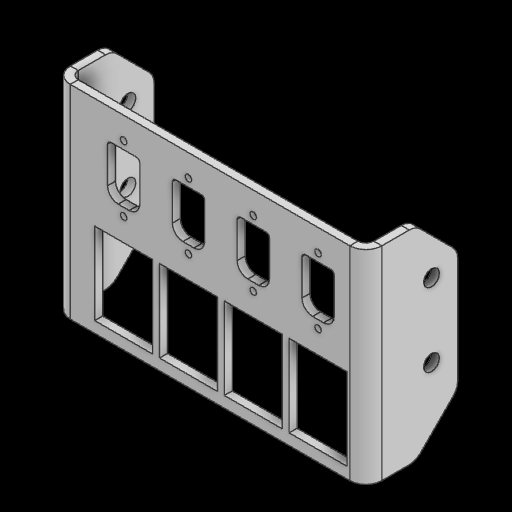
# Autodesk Inventor part: PowerHubFrontPanel
Saved by Autodesk Inventor 2025.2 (Build 292293000, 293)
## iProperties
Created: 2026-06-06
Part Number: PowerHubFrontPanel
Material: Generic
Document SubType Name: Sheet Metal
Designer: valer
Density: 1 g/cm^3
Appearance: Default
Sheet Metal Rule: Default
Author: valer
Autodesk Inventor part; units mm, degrees
ref_plane "YZ Plane" through (0, 0, 0) normal (1, 0, 0) x (0, 1, 0)
ref_plane "XZ Plane" through (0, 0, 0) normal (0, 1, 0) x (-1, 0, 0)
ref_plane "XY Plane" through (0, 0, 0) normal (0, 0, 1) x (1, 0, 0)
sketch "Base" plane through (0, 0, 0) normal (0, 0, 1) x (1, 0, 0)
  line L0 (-44.957, 34.75) -> (-28.957, 34.75) construction
  line L1 (-28.957, 34.75) -> (-28.957, 0.75) construction
  line L2 (-28.957, 0.75) -> (-44.957, 0.75) construction
  line L3 (-44.957, 0.75) -> (-44.957, 34.75) construction
  line L4 (-49.276, -3.25) -> (-24.638, -3.25) construction
  line L5 (-24.638, -3.25) -> (-24.638, -34.75) construction
  line L6 (-24.638, -34.75) -> (-49.276, -34.75) construction
  line L7 (-49.276, -34.75) -> (-49.276, -3.25) construction
  line L8 (-36.957, 0.75) -> (-36.957, -3.25) construction
  line L9 (-20.319, 0.75) -> (-20.319, 34.75) construction
  line L10 (-20.319, 34.75) -> (-4.319, 34.75) construction
  line L11 (-4.319, 34.75) -> (-4.319, 0.75) construction
  line L12 (-4.319, 0.75) -> (-20.319, 0.75) construction
  line L13 (-24.638, -3.25) -> (0, -3.25) construction
  line L14 (-24.638, -34.75) -> (-24.638, -3.25) construction
  line L15 (0, -3.25) -> (0, -34.75) construction
  line L16 (0, -34.75) -> (-24.638, -34.75) construction
  line L17 (4.319, 0.75) -> (4.319, 34.75) construction
  line L18 (4.319, 34.75) -> (20.319, 34.75) construction
  line L19 (20.319, 34.75) -> (20.319, 0.75) construction
  line L20 (20.319, 0.75) -> (4.319, 0.75) construction
  line L21 (0, -3.25) -> (24.638, -3.25) construction
  line L22 (0, -34.75) -> (0, -3.25) construction
  line L23 (24.638, -3.25) -> (24.638, -34.75) construction
  line L24 (24.638, -34.75) -> (0, -34.75) construction
  line L25 (28.957, 0.75) -> (28.957, 34.75) construction
  line L26 (28.957, 34.75) -> (44.957, 34.75) construction
  line L27 (44.957, 34.75) -> (44.957, 0.75) construction
  line L28 (44.957, 0.75) -> (28.957, 0.75) construction
  line L29 (24.638, -3.25) -> (49.276, -3.25) construction
  line L30 (24.638, -34.75) -> (24.638, -3.25) construction
  line L31 (49.276, -3.25) -> (49.276, -34.75) construction
  line L32 (49.276, -34.75) -> (24.638, -34.75) construction
  line L33 (-53.276, 38.75) -> (53.276, 38.75)
  line L34 (53.276, 38.75) -> (53.276, -38.75)
  line L35 (53.276, -38.75) -> (-53.276, -38.75)
  line L36 (-53.276, -38.75) -> (-53.276, 38.75)
  line L37 (0, -54.25) -> (0, 54.25)
  line L38 (-53.276, 38.75) -> (53.276, -38.75) construction
  point P0 (-12.319, 0.75)
  point P1 (-12.319, -3.25)
  point P2 (12.319, 0.75)
  point P3 (12.319, -3.25)
  point P4 (36.957, 0.75)
  point P5 (36.957, -3.25)
  point P6 (0, 0)
  point P7 (0, 0)
  dimension "d103" = 16
  dimension "d104" = 34
  dimension "d105" = 24.638
  dimension "d106" = 31.5
  dimension "d107" = 4
  dimension "d110" = 24.638
  dimension "d125" = 4
  dimension "d126" = 4
  dimension "d131" = 4
  dimension "d132" = 4
  measures "d103" distance of L0.start L0.end
  measures "d104" distance of L0.end L1.end
  measures "d105" distance of L5.end L6.end
  measures "d106" distance of L4.end L5.end
  measures "d107" distance between parallel lines of L4 L2
  measures "d110" distance of L2.end L9.start
  measures "d125" distance between parallel lines of L36 L7
  measures "d126" distance between parallel lines of L34 L31
  measures "d131" distance between parallel lines of L33 L26
  measures "d132" distance between parallel lines of L35 L32
extrude "Plate1" add sketch "Base" along normal blind 3.048
sketch "Instruments" plane through (0, 0, 0) normal (0, 0, -1) x (-1, 0, 0)
  circle A0 centre (-41.1741, 14.35) radius 2.5 construction
  circle A1 centre (-41.1741, 21.35) radius 2.5 construction
  arc A2 (-47.0741, 12.4) -> (-43.2741, 8.6) centre (-43.2741, 12.4) ccw construction
  line L0 (-43.2741, 8.6) -> (-39.0741, 8.6) construction
  arc A3 (-39.0741, 8.6) -> (-35.2741, 12.4) centre (-39.0741, 12.4) ccw construction
  line L1 (-35.2741, 12.4) -> (-35.2741, 26.1) construction
  arc A4 (-35.2741, 26.1) -> (-36.2741, 27.1) centre (-36.2741, 26.1) ccw construction
  line L2 (-36.2741, 27.1) -> (-46.0741, 27.1) construction
  arc A5 (-46.0741, 27.1) -> (-47.0741, 26.1) centre (-46.0741, 26.1) ccw construction
  line L3 (-47.0741, 26.1) -> (-47.0741, 12.4) construction
  circle A6 centre (-16.4741, 14.35) radius 2.5 construction
  circle A7 centre (-16.4741, 21.35) radius 2.5 construction
  arc A8 (-22.3741, 12.4) -> (-18.5741, 8.6) centre (-18.5741, 12.4) ccw construction
  line L4 (-18.5741, 8.6) -> (-14.3741, 8.6) construction
  arc A9 (-14.3741, 8.6) -> (-10.5741, 12.4) centre (-14.3741, 12.4) ccw construction
  line L5 (-10.5741, 12.4) -> (-10.5741, 26.1) construction
  arc A10 (-10.5741, 26.1) -> (-11.5741, 27.1) centre (-11.5741, 26.1) ccw construction
  line L6 (-11.5741, 27.1) -> (-21.3741, 27.1) construction
  arc A11 (-21.3741, 27.1) -> (-22.3741, 26.1) centre (-21.3741, 26.1) ccw construction
  line L7 (-22.3741, 26.1) -> (-22.3741, 12.4) construction
  circle A12 centre (8.2259, 14.35) radius 2.5 construction
  circle A13 centre (8.2259, 21.35) radius 2.5 construction
  arc A14 (2.3259, 12.4) -> (6.1259, 8.6) centre (6.1259, 12.4) ccw construction
  line L8 (6.1259, 8.6) -> (10.3259, 8.6) construction
  arc A15 (10.3259, 8.6) -> (14.1259, 12.4) centre (10.3259, 12.4) ccw construction
  line L9 (14.1259, 12.4) -> (14.1259, 26.1) construction
  arc A16 (14.1259, 26.1) -> (13.1259, 27.1) centre (13.1259, 26.1) ccw construction
  line L10 (13.1259, 27.1) -> (3.3259, 27.1) construction
  arc A17 (3.3259, 27.1) -> (2.3259, 26.1) centre (3.3259, 26.1) ccw construction
  line L11 (2.3259, 26.1) -> (2.3259, 12.4) construction
  circle A18 centre (32.9259, 14.35) radius 2.5 construction
  circle A19 centre (32.9259, 21.35) radius 2.5 construction
  arc A20 (27.0259, 12.4) -> (30.8259, 8.6) centre (30.8259, 12.4) ccw construction
  line L12 (30.8259, 8.6) -> (35.0259, 8.6) construction
  arc A21 (35.0259, 8.6) -> (38.8259, 12.4) centre (35.0259, 12.4) ccw construction
  line L13 (38.8259, 12.4) -> (38.8259, 26.1) construction
  arc A22 (38.8259, 26.1) -> (37.8259, 27.1) centre (37.8259, 26.1) ccw construction
  line L14 (37.8259, 27.1) -> (28.0259, 27.1) construction
  arc A23 (28.0259, 27.1) -> (27.0259, 26.1) centre (28.0259, 26.1) ccw construction
  line L15 (27.0259, 26.1) -> (27.0259, 12.4) construction
  line L16 (-47.8197, -7.45) -> (-34.5285, -7.45) construction
  line L17 (-34.5285, -7.45) -> (-34.5285, -30.45) construction
  line L18 (-34.5285, -30.45) -> (-47.8197, -30.45) construction
  line L19 (-47.8197, -30.45) -> (-47.8197, -7.45) construction
  line L20 (-30.3791, -3.6) -> (-51.9691, -3.6) construction
  line L21 (-51.9691, -3.6) -> (-51.9691, -34.3) construction
  line L22 (-51.9691, -34.3) -> (-30.3791, -34.3) construction
  line L23 (-30.3791, -34.3) -> (-30.3791, -3.6) construction
  line L24 (-23.1197, -7.45) -> (-9.8285, -7.45) construction
  line L25 (-9.8285, -7.45) -> (-9.8285, -30.45) construction
  line L26 (-9.8285, -30.45) -> (-23.1197, -30.45) construction
  line L27 (-23.1197, -30.45) -> (-23.1197, -7.45) construction
  line L28 (-5.6791, -3.6) -> (-27.2691, -3.6) construction
  line L29 (-27.2691, -3.6) -> (-27.2691, -34.3) construction
  line L30 (-27.2691, -34.3) -> (-5.6791, -34.3) construction
  line L31 (-5.6791, -34.3) -> (-5.6791, -3.6) construction
  line L32 (1.5803, -7.45) -> (14.8715, -7.45) construction
  line L33 (14.8715, -7.45) -> (14.8715, -30.45) construction
  line L34 (14.8715, -30.45) -> (1.5803, -30.45) construction
  line L35 (1.5803, -30.45) -> (1.5803, -7.45) construction
  line L36 (19.0209, -3.6) -> (-2.5691, -3.6) construction
  line L37 (-2.5691, -3.6) -> (-2.5691, -34.3) construction
  line L38 (-2.5691, -34.3) -> (19.0209, -34.3) construction
  line L39 (19.0209, -34.3) -> (19.0209, -3.6) construction
  line L40 (26.2803, -7.45) -> (39.5715, -7.45) construction
  line L41 (39.5715, -7.45) -> (39.5715, -30.45) construction
  line L42 (39.5715, -30.45) -> (26.2803, -30.45) construction
  line L43 (26.2803, -30.45) -> (26.2803, -7.45) construction
  line L44 (43.7209, -3.6) -> (22.1309, -3.6) construction
  line L45 (22.1309, -3.6) -> (22.1309, -34.3) construction
  line L46 (22.1309, -34.3) -> (43.7209, -34.3) construction
  line L47 (43.7209, -34.3) -> (43.7209, -3.6) construction
  line L48 (-46.0741, 27.35) -> (-36.2741, 27.35)
  arc A24 (-35.0241, 26.1) -> (-36.2741, 27.35) centre (-36.2741, 26.1) ccw
  line L49 (-35.0241, 26.1) -> (-35.0241, 12.4)
  arc A25 (-39.0741, 8.35) -> (-35.0241, 12.4) centre (-39.0741, 12.4) ccw
  line L50 (-39.0741, 8.35) -> (-43.2741, 8.35)
  arc A26 (-47.3241, 12.4) -> (-43.2741, 8.35) centre (-43.2741, 12.4) ccw
  line L51 (-47.3241, 12.4) -> (-47.3241, 26.1)
  arc A27 (-46.0741, 27.35) -> (-47.3241, 26.1) centre (-46.0741, 26.1) ccw
  line L52 (-21.3741, 27.35) -> (-11.5741, 27.35)
  arc A28 (-10.3241, 26.1) -> (-11.5741, 27.35) centre (-11.5741, 26.1) ccw
  line L53 (-10.3241, 26.1) -> (-10.3241, 12.4)
  arc A29 (-14.3741, 8.35) -> (-10.3241, 12.4) centre (-14.3741, 12.4) ccw
  line L54 (-14.3741, 8.35) -> (-18.5741, 8.35)
  arc A30 (-22.6241, 12.4) -> (-18.5741, 8.35) centre (-18.5741, 12.4) ccw
  line L55 (-22.6241, 12.4) -> (-22.6241, 26.1)
  arc A31 (-21.3741, 27.35) -> (-22.6241, 26.1) centre (-21.3741, 26.1) ccw
  line L56 (3.3259, 27.35) -> (13.1259, 27.35)
  arc A32 (14.3759, 26.1) -> (13.1259, 27.35) centre (13.1259, 26.1) ccw
  line L57 (14.3759, 26.1) -> (14.3759, 12.4)
  arc A33 (10.3259, 8.35) -> (14.3759, 12.4) centre (10.3259, 12.4) ccw
  line L58 (10.3259, 8.35) -> (6.1259, 8.35)
  arc A34 (2.0759, 12.4) -> (6.1259, 8.35) centre (6.1259, 12.4) ccw
  line L59 (2.0759, 12.4) -> (2.0759, 26.1)
  arc A35 (3.3259, 27.35) -> (2.0759, 26.1) centre (3.3259, 26.1) ccw
  line L60 (28.0259, 27.35) -> (37.8259, 27.35)
  arc A36 (39.0759, 26.1) -> (37.8259, 27.35) centre (37.8259, 26.1) ccw
  line L61 (39.0759, 26.1) -> (39.0759, 12.4)
  arc A37 (35.0259, 8.35) -> (39.0759, 12.4) centre (35.0259, 12.4) ccw
  line L62 (35.0259, 8.35) -> (30.8259, 8.35)
  arc A38 (26.7759, 12.4) -> (30.8259, 8.35) centre (30.8259, 12.4) ccw
  line L63 (26.7759, 12.4) -> (26.7759, 26.1)
  arc A39 (28.0259, 27.35) -> (26.7759, 26.1) centre (28.0259, 26.1) ccw
  line L64 (43.9709, -3.35) -> (21.8809, -3.35)
  line L65 (21.8809, -3.35) -> (21.8809, -34.55)
  line L66 (21.8809, -34.55) -> (43.9709, -34.55)
  line L67 (43.9709, -34.55) -> (43.9709, -3.35)
  line L68 (-2.8191, -3.35) -> (19.2709, -3.35)
  line L69 (19.2709, -3.35) -> (19.2709, -34.55)
  line L70 (19.2709, -34.55) -> (-2.8191, -34.55)
  line L71 (-2.8191, -34.55) -> (-2.8191, -3.35)
  line L72 (-27.5191, -3.35) -> (-5.4291, -3.35)
  line L73 (-5.4291, -3.35) -> (-5.4291, -34.55)
  line L74 (-5.4291, -34.55) -> (-27.5191, -34.55)
  line L75 (-27.5191, -34.55) -> (-27.5191, -3.35)
  line L76 (-52.2191, -3.35) -> (-30.1291, -3.35)
  line L77 (-30.1291, -3.35) -> (-30.1291, -34.55)
  line L78 (-30.1291, -34.55) -> (-52.2191, -34.55)
  line L79 (-52.2191, -34.55) -> (-52.2191, -3.35)
  circle A40 centre (32.9259, 30.35) radius 1.55 construction
  circle A41 centre (32.9259, 5.35) radius 1.55 construction
  circle A42 centre (8.2259, 5.35) radius 1.55 construction
  circle A43 centre (8.2259, 30.35) radius 1.55 construction
  circle A44 centre (-16.4741, 30.35) radius 1.55 construction
  circle A45 centre (-16.4741, 5.35) radius 1.55 construction
  circle A46 centre (-41.1741, 30.35) radius 1.55 construction
  circle A47 centre (-41.1741, 5.35) radius 1.55 construction
  circle A48 centre (-41.1741, 30.35) radius 1.25
  circle A49 centre (-16.4741, 30.35) radius 1.25
  circle A50 centre (8.2259, 30.35) radius 1.25
  circle A51 centre (32.9259, 30.35) radius 1.25
  circle A52 centre (-41.1741, 5.35) radius 1.25
  circle A53 centre (-16.4741, 5.35) radius 1.25
  circle A54 centre (8.2259, 5.35) radius 1.25
  circle A55 centre (32.9259, 5.35) radius 1.25
  point P0 (0, 0)
  dimension "d134" = 0.25
  dimension "d135" = 0.25
  dimension "d136" = 0.25
  dimension "d137" = 0.25
  dimension "d138" = 0.25
  dimension "d139" = 0.25
  dimension "d140" = 0.25
  dimension "d141" = 0.25
  dimension "d144" = 2.5
  constraints: 64 end point, 32 point on circle, 24 centre point, 8 coincident, 7 equal radius, 40 other
  measures "d134" distance between parallel lines of L2 L48
  measures "d135" distance between parallel lines of L6 L52
  measures "d136" distance between parallel lines of L10 L56
  measures "d137" distance between parallel lines of L14 L60
  measures "d138" distance between parallel lines of L47 L67
  measures "d139" distance between parallel lines of L36 L68
  measures "d140" distance between parallel lines of L28 L72
  measures "d141" distance between parallel lines of L20 L76
  measures "d144" diameter of A48
extrude "InstrumentsFeature" cut sketch "Instruments" against normal blind 3.048
sketch "Sketch10" plane through (-56.324, 38.75, -3.048) normal (-1, 0, 0) x (0, -1, 0)
  line L0 (77.5, 0) -> (0, 0)
  line L1 (0, 0) -> (0, -28.904)
  line L2 (0, -28.904) -> (77.5, -28.904)
  line L3 (77.5, -28.904) -> (77.5, 0)
  constraints: 6 end point, 1 horizontal, 1 perpendicular, 1 vertical
edge flange "MountFeature" height 35 angle 90 thickness 3.048 bend radius 3.048 thickness toward (-1, 0, 0) relief straight relief width 3.048 relief depth 1.524 corner gap 3.048 corner form 0 edges at (-53.276, 0, 0) (53.276, 0, 0) wall of the first edge with corners at (-56.324, -38.75, -3.048) (-56.324, 38.75, -3.048) (-56.324, 38.75, -31.952) (-56.324, -38.75, -31.952)
bend "Bend1"
corner "Corner1"
chamfer "MountChamfersFeature" distance 16 angle 45 4 edges at (57.848, -38.75, -31.952) (-57.848, -38.75, -31.952) (57.848, 38.75, -31.952) (-57.848, 38.75, -31.952)
fillet "MountFilletsFeature" radius 6 8 edges at (57.848, -38.75, -15.952) (57.848, -22.75, -31.952) (-57.848, -38.75, -15.952) (-57.848, -22.75, -31.952) (57.848, 22.75, -31.952) (57.848, 38.75, -15.952) (-57.848, 22.75, -31.952) (-57.848, 38.75, -15.952)
sketch "Sketch11" plane through (-59.372, -38.75, -3.048) normal (-1, 0, 0) x (0, 0, 1)
  circle A0 centre (-18.904, 29.5122) radius 3
  circle A1 centre (-18.904, 57.5122) radius 3
  arc A2 (-16.7827, 31.6335) -> (-21.0253, 27.3909) centre (-18.904, 29.5122) ccw projected
  arc A3 (-16.7827, 59.6335) -> (-21.0253, 55.3909) centre (-18.904, 57.5122) ccw projected
  point P0 (3.048, 38.75)
  constraints: 1 centre point, 1 concentric, 3 other
extrude "Cut2" cut sketch "Sketch11" against normal through all
body "Solid3"
